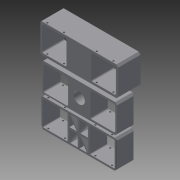
# Autodesk Inventor part: Part2
Saved by Autodesk Inventor 2015 (Build 190159000, 159)
## iProperties
Created: 2015-03-12
Part Number: Part2
Material: Generic
Document SubType Name: Modeling
Designer: Vladimir
Density: 1 g/cm^3
Appearance: Default
Author: Vladimir
Autodesk Inventor part; units mm, degrees
ref_plane "YZ Plane" through (0, 0, 0) normal (1, 0, 0) x (0, 1, 0)
ref_plane "XZ Plane" through (0, 0, 0) normal (0, 1, 0) x (-1, 0, 0)
ref_plane "XY Plane" through (0, 0, 0) normal (0, 0, 1) x (1, 0, 0)
sketch "Sketch2" plane through (0, 0, 0) normal (0, 0, 1) x (1, 0, 0)
  line L0 (-52.8, 0) -> (-52.8, 26.8)
  line L1 (-25, 0) -> (-49.8, 0)
  line L2 (-50.8, 1) -> (-50.8, 25.8)
  line L3 (-49.8, 26.8) -> (-25, 26.8)
  line L4 (-24, 25.8) -> (-24, 1)
  line L5 (1, 0) -> (25.8, 0)
  line L6 (26.8, 1) -> (26.8, 25.8)
  line L7 (25.8, 26.8) -> (1, 26.8)
  line L8 (0, 25.8) -> (0, 1)
  line L9 (28.8, 0) -> (28.8, 26.8)
  line L10 (-14, 12.4) -> (-22, 1)
  line L11 (-21, 0) -> (-13, 11.4)
  line L12 (-22, 12.4) -> (-22, 1)
  line L13 (-21, 0) -> (-13, 0)
  line L14 (-13, 11.4) -> (-13, 0)
  line L15 (-14, 12.4) -> (-22, 12.4)
  line L16 (-10.0871, 14.4487) -> (-2, 25.7407)
  line L17 (-10.0871, 14.4487) -> (-2, 14.4487)
  line L18 (-2.9547, 26.8) -> (-11.0272, 15.5285)
  line L19 (-11.0272, 26.8) -> (-11.0272, 15.5285)
  line L20 (-2.9547, 26.8) -> (-11.0272, 26.8)
  line L21 (-2, 25.7407) -> (-2, 14.4487)
  line L22 (-50.8, -2) -> (26.8, -2)
  line L23 (-50.8, 28.8) -> (26.8, 28.8)
  line L24 (-10.0272, 12.4) -> (-2, 1)
  line L25 (-3, 0) -> (-11.0272, 11.4)
  line L26 (-3, 0) -> (-11.0272, 0)
  line L27 (-2, 1) -> (-2, 12.4)
  line L28 (-11.0272, 11.4) -> (-11.0272, 0)
  line L29 (-10.0272, 12.4) -> (-2, 12.4)
  line L30 (-13, 15.4487) -> (-21, 26.8)
  line L31 (-22, 25.8) -> (-14, 14.4487)
  line L32 (-13, 26.8) -> (-21, 26.8)
  line L33 (-22, 25.8) -> (-22, 14.4487)
  line L34 (-13, 26.8) -> (-13, 15.4487)
  line L35 (-14, 14.4487) -> (-22, 14.4487)
  arc A0 (1, 26.8) -> (0, 25.8) centre (1, 25.8) ccw
  arc A1 (0, 1) -> (1, 0) centre (1, 1) ccw
  arc A2 (25.8, 0) -> (26.8, 1) centre (25.8, 1) ccw
  arc A3 (26.8, 25.8) -> (25.8, 26.8) centre (25.8, 25.8) ccw
  arc A4 (-49.8, 26.8) -> (-50.8, 25.8) centre (-49.8, 25.8) ccw
  arc A5 (-24, 25.8) -> (-25, 26.8) centre (-25, 25.8) ccw
  arc A6 (-25, 0) -> (-24, 1) centre (-25, 1) ccw
  arc A7 (-50.8, 1) -> (-49.8, 0) centre (-49.8, 1) ccw
  line L36 (26.8, -2) -> (28.8, 0)
  line L37 (26.8, 28.8) -> (28.8, 26.8)
  line L38 (-52.8, 0) -> (-50.8, -2)
  line L39 (-50.8, 28.8) -> (-52.8, 26.8)
  point P0 (0, 0)
  point P1 (-52.8, 28.8)
  point P2 (-52.8, -2)
  point P3 (-24, 0)
  point P4 (-50.8, 26.8)
  point P5 (-50.8, 0)
  point P6 (-24, 26.8)
  point P7 (26.8, 26.8)
  point P8 (0, 26.8)
  point P9 (28.8, 28.8)
  point P10 (28.8, -2)
  dimension "d11" = 30.8
  dimension "d12" = 26.8
  dimension "d13" = 26.8
  dimension "d14" = 26.8
  dimension "d34" = 2
  dimension "d35" = 1.393
  dimension "d36" = 3
  dimension "d40" = 13.9269
  dimension "d41" = 1.393
  dimension "d45" = 2
  dimension "d46" = 2
  dimension "d47" = 2
  dimension "d48" = 81.6
  dimension "d49" = 2
  dimension "d50" = 11.2715
  dimension "d68" = 1
  dimension "d69" = 1
  dimension "d70" = 1
  dimension "d71" = 1
  dimension "d72" = 1
  dimension "d73" = 1
  dimension "d74" = 1
  dimension "d75" = 1
  dimension "d76" = 2
  dimension "d77" = 2
  dimension "d78" = 2
  dimension "d79" = 2
  dimension "d80" = 2
  dimension "d81" = 2
  dimension "d82" = 2
  dimension "d83" = 2
  constraints: 80 end point, 21 point on line, 16 point on circle, 16 tangent, 9 perpendicular, 8 centre point, 7 vertical, 6 horizontal, 6 parallel
  measures "d11" distance of point (-52.8, -2) point (-52.8, 28.8)
  measures "d12" distance of point (-50.8, 26.8) point (-24, 26.8)
  measures "d13" distance of point (-50.8, 0) point (-50.8, 26.8)
  measures "d14" distance of point (0, 26.8) point (26.8, 26.8)
  measures "d34" distance from line of L4 L12.start
  measures "d35" distance between parallel lines of L11 L10
  measures "d36" distance of point (-24, 0) L11.start
  measures "d40" distance of L11.start L11.end
  measures "d41" distance between parallel lines of L16 L18
  measures "d45" distance between parallel lines of L8 L21
  measures "d46" distance between parallel lines of L9 L6
  measures "d47" distance between parallel lines of L0 L2
  measures "d48" distance of point (-52.8, 28.8) point (28.8, 28.8)
  measures "d49" distance between parallel lines of L20 L23
  measures "d50" distance of L19.start L18.end
  measures "d68" radius of A0
  measures "d69" radius of A1
  measures "d70" radius of A2
  measures "d71" radius of A3
  measures "d72" radius of A4
  measures "d73" radius of A5
  measures "d74" radius of A6
  measures "d75" radius of A7
  measures "d76" distance of L22.end point (28.8, -2)
  measures "d77" distance of L9.start point (28.8, -2)
  measures "d78" distance of L23.end point (28.8, 28.8)
  measures "d79" distance of L9.end point (28.8, 28.8)
  measures "d80" distance of L0.start point (-52.8, -2)
  measures "d81" distance of L22.start point (-52.8, -2)
  measures "d82" distance of L23.start point (-52.8, 28.8)
  measures "d83" distance of L0.end point (-52.8, 28.8)
extrude "Extrusion1" add sketch "Sketch2" along normal blind 18.7
sketch "Sketch3" plane through (-50.8, 28.8, 0) normal (0, 1, 0) x (1, 0, 0)
  line L0 (-2, 0) -> (79.6, 0)
  line L1 (79.6, 0) -> (79.6, -18.7)
  line L2 (79.6, -18.7) -> (-2, -18.7)
  line L3 (-2, -18.7) -> (-2, 0)
  circle A0 centre (4.4, -17) radius 0.8
  circle A1 centre (22.4, -17) radius 0.8
  line L4 (0, 0) -> (-2, 0)
  line L5 (-2, 0) -> (-2, -18.7)
  line L6 (-2, -18.7) -> (0, -18.7)
  line L7 (0, -18.7) -> (0, 0)
  line L8 (0, -18.7) -> (0.2, -18.7)
  line L9 (0.2, -18.7) -> (0.2, 0)
  line L10 (0.2, 0) -> (0, 0)
  line L11 (0, 0) -> (0, -18.7)
  line L12 (77.6, 0) -> (0, 0) projected
  line L13 (0.2, -18.7) -> (26.6, -18.7)
  line L14 (26.6, -18.7) -> (26.6, 0)
  line L15 (26.6, 0) -> (0.2, 0)
  line L16 (0.2, 0) -> (0.2, -18.7)
  line L17 (79.6, 0) -> (77.4, 0)
  line L18 (77.4, 0) -> (77.4, -18.7)
  line L19 (77.4, -18.7) -> (79.6, -18.7)
  line L20 (79.6, -18.7) -> (79.6, 0)
  circle A2 centre (73.2, -17) radius 0.8
  circle A3 centre (55.2, -17) radius 0.8
  point P0 (50.8, 0)
  dimension "d98" = 1.6
  dimension "d99" = 1.6
  dimension "d115" = 2.2
  dimension "d116" = 1.6
  dimension "d117" = 1.6
  dimension "d118" = 18
  dimension "d119" = 4.2
  dimension "d120" = 1.7
  dimension "d121" = 1.7
  constraints: 40 end point, 10 parallel, 5 horizontal, 5 perpendicular, 4 centre point, 4 point on line
  measures "d98" diameter of A0
  measures "d99" diameter of A1
  measures "d115" distance of L19.end L18.end
  measures "d116" diameter of A2
  measures "d117" diameter of A3
  measures "d118" distance of A2.centre A3.centre
  measures "d119" distance from line of L18 A2.centre
  measures "d120" distance from line of L2 A3.centre
  measures "d121" distance from line of L2 A2.centre
hole "Hole3" at (-52.8, 28.8, 0) at (28.8, 28.8, 18.7) at (-46.4, 28.8, 17) at (-28.4, 28.8, 17) at (4.4, 28.8, 17) at (22.4, 28.8, 17) direction (0, -1, 0) diameter 1.9 end through all
move or copy body "Move Body2" bodies to move or copy 1 copy no translate (0, 35, 0)
sketch "Sketch4" plane through (-50.8, 63.8, 18.7) normal (0, 0, 1) x (1, 0, 0)
  line L0 (-1.385, 4.7525) -> (-1.385, 31.5525)
  line L1 (25.815, 4.2525) -> (2.115, 4.2525)
  line L2 (0.615, 5.7525) -> (0.615, 29.4525)
  line L3 (2.115, 30.9525) -> (25.815, 30.9525)
  line L4 (27.315, 29.4525) -> (27.315, 5.7525)
  line L5 (53.015, 4.8525) -> (76.715, 4.8525)
  line L6 (78.215, 6.3525) -> (78.215, 30.0525)
  line L7 (76.715, 31.5525) -> (53.015, 31.5525)
  line L8 (51.515, 30.0525) -> (51.515, 6.3525)
  line L9 (80.215, 4.7525) -> (80.215, 31.5525)
  line L10 (0.615, 2.7525) -> (78.215, 2.7525)
  line L11 (0.615, 33.5525) -> (78.215, 33.5525)
  arc A0 (53.015, 31.5525) -> (51.515, 30.0525) centre (53.015, 30.0525) ccw
  arc A1 (51.515, 6.3525) -> (53.015, 4.8525) centre (53.015, 6.3525) ccw
  arc A2 (76.715, 4.8525) -> (78.215, 6.3525) centre (76.715, 6.3525) ccw
  arc A3 (78.215, 30.0525) -> (76.715, 31.5525) centre (76.715, 30.0525) ccw
  arc A4 (2.115, 30.9525) -> (0.615, 29.4525) centre (2.115, 29.4525) ccw
  arc A5 (27.315, 29.4525) -> (25.815, 30.9525) centre (25.815, 29.4525) ccw
  arc A6 (25.815, 4.2525) -> (27.315, 5.7525) centre (25.815, 5.7525) ccw
  arc A7 (0.615, 5.7525) -> (2.115, 4.2525) centre (2.115, 5.7525) ccw
  line L12 (78.215, 2.7525) -> (80.215, 4.7525)
  line L13 (78.215, 33.5525) -> (80.215, 31.5525)
  line L14 (-1.385, 4.7525) -> (0.615, 2.7525)
  line L15 (0.615, 33.5525) -> (-1.385, 31.5525)
  circle A8 centre (39.415, 18.1525) radius 6.0399
  point P0 (50.8, -63.8)
  point P1 (51.415, 4.7525)
  point P2 (-1.385, 33.5525)
  point P3 (-1.385, 2.7525)
  point P4 (27.315, 4.2525)
  point P5 (0.615, 30.9525)
  point P6 (0.615, 4.2525)
  point P7 (27.315, 30.9525)
  point P8 (78.215, 31.5525)
  point P9 (51.515, 31.5525)
  point P10 (80.215, 33.5525)
  point P11 (80.215, 2.7525)
  dimension "d132" = 30.8
  dimension "d133" = 26.7
  dimension "d134" = 26.7
  dimension "d135" = 26.7
  dimension "d142" = 2
  dimension "d143" = 2
  dimension "d144" = 81.6
  dimension "d147" = 1.5
  dimension "d148" = 1.5
  dimension "d149" = 1.5
  dimension "d150" = 1.5
  dimension "d151" = 1.5
  dimension "d152" = 1.5
  dimension "d153" = 1.5
  dimension "d154" = 1.5
  dimension "d155" = 2
  dimension "d156" = 2
  dimension "d157" = 2
  dimension "d158" = 2
  dimension "d159" = 2
  dimension "d160" = 2
  dimension "d161" = 2
  dimension "d162" = 2
  dimension "d164" = 26.7
  dimension "d165" = 15.4
  dimension "d205" = 24.2
  dimension "d206" = 28.7
  constraints: 32 end point, 20 point on line, 16 point on circle, 16 tangent, 9 centre point, 4 horizontal, 4 parallel, 2 perpendicular
  measures "d132" distance of point (-1.385, 2.752) point (-1.385, 33.552)
  measures "d133" distance of point (0.615, 30.952) point (27.315, 30.952)
  measures "d134" distance of point (0.615, 4.252) point (0.615, 30.952)
  measures "d135" distance of point (51.515, 31.552) point (78.215, 31.552)
  measures "d142" distance between parallel lines of L9 L6
  measures "d143" distance between parallel lines of L0 L2
  measures "d144" distance of point (-1.385, 33.552) point (80.215, 33.552)
  measures "d147" radius of A0
  measures "d148" radius of A1
  measures "d149" radius of A2
  measures "d150" radius of A3
  measures "d151" radius of A4
  measures "d152" radius of A5
  measures "d153" radius of A6
  measures "d154" radius of A7
  measures "d155" distance of L10.end point (80.215, 2.752)
  measures "d156" distance of L9.start point (80.215, 2.752)
  measures "d157" distance of L11.end point (80.215, 33.552)
  measures "d158" distance of L9.end point (80.215, 33.552)
  measures "d159" distance of L0.start point (-1.385, 2.752)
  measures "d160" distance of L10.start point (-1.385, 2.752)
  measures "d161" distance of L11.start point (-1.385, 33.552)
  measures "d162" distance of L0.end point (-1.385, 33.552)
  measures "d164" distance between parallel lines of L5 L7
  measures "d165" distance from line of L10 A8.centre
  measures "d205" distance between parallel lines of L8 L4
  measures "d206" distance between parallel lines of L0 L4
sketch "Sketch5" plane through (-50.8, 63.8, 18.7) normal (0, 0, 1) x (1, 0, 0)
  line L0 (-3.4931, 39.9306) -> (-3.4931, 67.5306)
  line L1 (24.1569, 40.3806) -> (0.5069, 40.3806)
  line L2 (-0.9931, 41.8806) -> (-0.9931, 65.5306)
  line L3 (0.5069, 67.0306) -> (24.1569, 67.0306)
  line L4 (25.6569, 65.5306) -> (25.6569, 41.8806)
  line L5 (53.8569, 40.3806) -> (77.5069, 40.3806)
  line L6 (79.0069, 41.8806) -> (79.0069, 65.5306)
  line L7 (77.5069, 67.0306) -> (53.8569, 67.0306)
  line L8 (52.3569, 65.5306) -> (52.3569, 41.8806)
  line L9 (81.5069, 39.9306) -> (81.5069, 67.5306)
  line L10 (-1.4931, 37.9306) -> (79.5069, 37.9306)
  line L11 (-1.4931, 69.5306) -> (79.5069, 69.5306)
  arc A0 (53.8569, 67.0306) -> (52.3569, 65.5306) centre (53.8569, 65.5306) ccw
  arc A1 (52.3569, 41.8806) -> (53.8569, 40.3806) centre (53.8569, 41.8806) ccw
  arc A2 (77.5069, 40.3806) -> (79.0069, 41.8806) centre (77.5069, 41.8806) ccw
  arc A3 (79.0069, 65.5306) -> (77.5069, 67.0306) centre (77.5069, 65.5306) ccw
  arc A4 (0.5069, 67.0306) -> (-0.9931, 65.5306) centre (0.5069, 65.5306) ccw
  arc A5 (25.6569, 65.5306) -> (24.1569, 67.0306) centre (24.1569, 65.5306) ccw
  arc A6 (24.1569, 40.3806) -> (25.6569, 41.8806) centre (24.1569, 41.8806) ccw
  arc A7 (-0.9931, 41.8806) -> (0.5069, 40.3806) centre (0.5069, 41.8806) ccw
  line L12 (79.5069, 37.9306) -> (81.5069, 39.9306)
  line L13 (79.5069, 69.5306) -> (81.5069, 67.5306)
  line L14 (-3.4931, 39.9306) -> (-1.4931, 37.9306)
  line L15 (-1.4931, 69.5306) -> (-3.4931, 67.5306)
  point P0 (50.8, -63.8)
  point P1 (50.8, -63.8)
  point P2 (49.3069, 39.9306)
  point P3 (-3.4931, 69.5306)
  point P4 (-3.4931, 37.9306)
  point P5 (25.6569, 40.3806)
  point P6 (-0.9931, 67.0306)
  point P7 (-0.9931, 40.3806)
  point P8 (25.6569, 67.0306)
  point P9 (79.0069, 67.0306)
  point P10 (52.3569, 67.0306)
  point P11 (81.5069, 69.5306)
  point P12 (81.5069, 37.9306)
  dimension "d166" = 31.6
  dimension "d167" = 26.65
  dimension "d168" = 26.65
  dimension "d169" = 26.65
  dimension "d170" = 2.5
  dimension "d171" = 2.5
  dimension "d172" = 85
  dimension "d173" = 1.5
  dimension "d174" = 1.5
  dimension "d175" = 1.5
  dimension "d176" = 1.5
  dimension "d177" = 1.5
  dimension "d178" = 1.5
  dimension "d179" = 1.5
  dimension "d180" = 1.5
  dimension "d181" = 2
  dimension "d182" = 2
  dimension "d183" = 2
  dimension "d184" = 2
  dimension "d185" = 2
  dimension "d186" = 2
  dimension "d187" = 2
  dimension "d188" = 2
  dimension "d189" = 26.65
  dimension "d191" = 2.5
  dimension "d192" = 2.5
  dimension "d193" = 2.45
  dimension "d228" = 29.15
  constraints: 32 end point, 20 point on line, 16 point on circle, 16 tangent, 8 centre point, 4 horizontal, 4 parallel, 2 perpendicular
  measures "d166" distance of point (-3.493, 37.931) point (-3.493, 69.531)
  measures "d167" distance of point (-0.993, 67.031) point (25.657, 67.031)
  measures "d168" distance of point (-0.993, 40.381) point (-0.993, 67.031)
  measures "d169" distance of point (52.357, 67.031) point (79.007, 67.031)
  measures "d170" distance between parallel lines of L9 L6
  measures "d171" distance between parallel lines of L0 L2
  measures "d172" distance of point (-3.493, 69.531) point (81.507, 69.531)
  measures "d173" radius of A0
  measures "d174" radius of A1
  measures "d175" radius of A2
  measures "d176" radius of A3
  measures "d177" radius of A4
  measures "d178" radius of A5
  measures "d179" radius of A6
  measures "d180" radius of A7
  measures "d181" distance of L10.end point (81.507, 37.931)
  measures "d182" distance of L9.start point (81.507, 37.931)
  measures "d183" distance of L11.end point (81.507, 69.531)
  measures "d184" distance of L9.end point (81.507, 69.531)
  measures "d185" distance of L0.start point (-3.493, 37.931)
  measures "d186" distance of L10.start point (-3.493, 37.931)
  measures "d187" distance of L11.start point (-3.493, 69.531)
  measures "d188" distance of L0.end point (-3.493, 69.531)
  measures "d189" distance between parallel lines of L5 L7
  measures "d191" distance between parallel lines of L11 L3
  measures "d192" distance between parallel lines of L11 L7
  measures "d193" distance between parallel lines of L10 L1
  measures "d228" distance between parallel lines of L0 L4
extrude "Extrusion2" add sketch "Sketch4" against normal blind 18.7
extrude "Extrusion3" add sketch "Sketch5" against normal blind 24
sketch "extrusion 2 holes" plane through (-50.185, 97.3525, 18.7) normal (0, 1, 0) x (1, 0, 0)
  line L0 (79.6, 18.7) -> (-2, 18.7)
  line L1 (-2, 18.7) -> (-2, 0)
  line L2 (-2, 0) -> (79.6, 0)
  line L3 (79.6, 0) -> (79.6, 18.7)
  line L4 (79.6, 18.7) -> (77.45, 18.7)
  line L5 (77.45, 18.7) -> (77.45, 0)
  line L6 (77.45, 0) -> (79.6, 0)
  line L7 (79.6, 0) -> (79.6, 18.7)
  line L8 (77.45, 18.7) -> (51.05, 18.7)
  line L9 (51.05, 18.7) -> (51.05, 0)
  line L10 (51.05, 0) -> (77.45, 0)
  line L11 (77.45, 0) -> (77.45, 18.7)
  line L12 (1.5, 0) -> (0, 0) projected
  line L13 (-2, 18.7) -> (0.15, 18.7)
  line L14 (0.15, 18.7) -> (0.15, 0)
  line L15 (0.15, 0) -> (-2, 0)
  line L16 (-2, 0) -> (-2, 18.7)
  line L17 (0.15, 18.7) -> (26.55, 18.7)
  line L18 (26.55, 18.7) -> (26.55, 0)
  line L19 (26.55, 0) -> (0.15, 0)
  line L20 (0.15, 0) -> (0.15, 18.7)
  line L21 (77.6, 0) -> (0, 0) projected
  line L22 (0, 18.7) -> (77.6, 18.7) projected
  line L23 (50.7639, 0) -> (26.757, 0)
  line L24 (26.757, 0) -> (26.757, 18.7)
  line L25 (26.757, 18.7) -> (50.7639, 18.7)
  line L26 (51.05, 0) -> (50.9, 0)
  line L27 (50.9, 0) -> (50.9, 18.7)
  line L28 (50.9, 18.7) -> (51.05, 18.7)
  line L29 (51.05, 18.7) -> (51.05, 0)
  circle A0 centre (73.25, 17) radius 0.95
  circle A1 centre (55.25, 17) radius 0.95
  circle A2 centre (22.35, 17) radius 0.95
  circle A3 centre (4.35, 17) radius 0.95
  point P0 (50.185, 18.7)
  dimension "d201" = 2.15
  dimension "d202" = 26.4
  dimension "d203" = 2.15
  dimension "d204" = 26.4
  dimension "d207" = 0.15
  dimension "d208" = 28.7
  dimension "d209" = 1.9
  dimension "d210" = 1.9
  dimension "d211" = 18
  dimension "d212" = 4.2
  dimension "d213" = 1.7
  dimension "d214" = 1.7
  dimension "d215" = 1.9
  dimension "d216" = 1.9
  dimension "d217" = 18
  dimension "d218" = 4.2
  dimension "d219" = 1.7
  dimension "d220" = 1.7
  constraints: 54 end point, 13 parallel, 7 horizontal, 7 perpendicular, 6 point on line, 4 centre point
  measures "d201" distance of L6.end L5.end
  measures "d202" distance of L10.end L9.end
  measures "d203" distance of L14.end L15.end
  measures "d204" distance of L18.end L19.end
  measures "d207" distance of L27.end L28.end
  measures "d208" distance between parallel lines of L27 L7
  measures "d209" diameter of A1
  measures "d210" diameter of A0
  measures "d211" distance of A1.centre A0.centre
  measures "d212" distance from line of L5 A0.centre
  measures "d213" distance from line of L0 A1.centre
  measures "d214" distance from line of A0.centre L8
  measures "d215" diameter of A2
  measures "d216" diameter of A3
  measures "d217" distance of A3.centre A2.centre
  measures "d218" distance from line of A2.centre L18
  measures "d219" distance from line of L17 A2.centre
  measures "d220" distance from line of L0 A3.centre
hole "Hole4" at (29.415, 97.3525, 0) at (-52.185, 97.3525, 18.7) at (-27.835, 97.3525, 1.7) at (-45.835, 97.3525, 1.7) at (5.065, 97.3525, 1.7) at (23.065, 97.3525, 1.7) direction (0, -1, 0) diameter 1.9 end through all
sketch "Sketch7" plane through (-52.2931, 101.7306, 18.7) normal (0, -1, 0) x (1, 0, 0)
  line L0 (-2, 0) -> (83, 0)
  line L1 (83, 0) -> (83, -24)
  line L2 (83, -24) -> (-2, -24)
  line L3 (-2, -24) -> (-2, 0)
  line L4 (0, -24) -> (81, -24) projected
  line L5 (83, 0) -> (80.375, 0)
  line L6 (80.375, 0) -> (80.375, -24)
  line L7 (80.375, -24) -> (83, -24)
  line L8 (83, -24) -> (83, 0)
  line L9 (81, 0) -> (0, 0) projected
  line L10 (80.375, -24) -> (53.975, -24)
  line L11 (53.975, -24) -> (53.975, 0)
  line L12 (53.975, 0) -> (80.375, 0)
  line L13 (80.375, 0) -> (80.375, -24)
  circle A0 centre (76.175, -1.7) radius 0.95
  circle A1 centre (58.175, -1.7) radius 0.95
  line L14 (-2, -24) -> (0.625, -24)
  line L15 (0.625, -24) -> (0.625, 0)
  line L16 (0.625, 0) -> (-2, 0)
  line L17 (-2, 0) -> (-2, -24)
  line L18 (0.625, 0) -> (27.025, 0)
  line L19 (27.025, 0) -> (27.025, -24)
  line L20 (27.025, -24) -> (0.625, -24)
  line L21 (0.625, -24) -> (0.625, 0)
  circle A2 centre (22.825, -1.7) radius 0.95
  circle A3 centre (4.825, -1.7) radius 0.95
  point P0 (52.2931, -18.7)
  dimension "d229" = 2.625
  dimension "d230" = 26.4
  dimension "d231" = 29.025
  dimension "d232" = 1.9
  dimension "d233" = 1.9
  dimension "d234" = 18
  dimension "d235" = 4.2
  dimension "d236" = 4.2
  dimension "d237" = 1.7
  dimension "d238" = 2.625
  dimension "d239" = 26.4
  dimension "d240" = 1.9
  dimension "d241" = 1.9
  dimension "d242" = 18
  dimension "d243" = 4.2
  dimension "d244" = 4.2
  dimension "d245" = 1.7
  constraints: 40 end point, 10 parallel, 5 horizontal, 5 perpendicular, 4 centre point, 4 point on line
  measures "d229" distance of L7.end L6.end
  measures "d230" distance of L11.end L12.end
  measures "d231" distance between parallel lines of L11 L1
  measures "d232" diameter of A1
  measures "d233" diameter of A0
  measures "d234" distance of A1.centre A0.centre
  measures "d235" distance from line of L6 A0.centre
  measures "d236" distance from line of L11 A1.centre
  measures "d237" distance from line of L12 A1.centre
  measures "d238" distance of L16.end L15.end
  measures "d239" distance of L19.end L20.end
  measures "d240" diameter of A2
  measures "d241" diameter of A3
  measures "d242" distance of A3.centre A2.centre
  measures "d243" distance from line of L19 A2.centre
  measures "d244" distance from line of L15 A3.centre
  measures "d245" distance from line of L9 A3.centre
hole "Hole5" at (-54.2931, 101.7306, 18.7) at (23.8819, 101.7306, 17) at (5.8819, 101.7306, 17) at (-29.4681, 101.7306, 17) at (-47.4681, 101.7306, 17) direction (0, 1, 0) diameter 1.9 end through all
body "Solid1"
